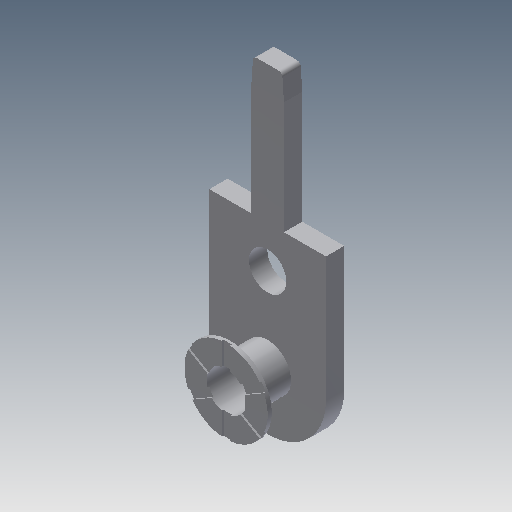
# Autodesk Inventor part: Part4_panel pot
Saved by Autodesk Inventor 2020 (Build 240168000, 168)
## iProperties
Created: 2016-08-22
Part Number: Part4_panel pot
Material: Generic
Document SubType Name: Modeling
Designer: Tom
Density: 1 g/cm^3
Appearance: Default
Author: Tom
Autodesk Inventor part; units mm, degrees
ref_plane "YZ Plane" through (0, 0, 0) normal (1, 0, 0) x (0, 1, 0)
ref_plane "XZ Plane" through (0, 0, 0) normal (0, 1, 0) x (-1, 0, 0)
ref_plane "XY Plane" through (0, 0, 0) normal (0, 0, 1) x (1, 0, 0)
sketch "Sketch1" plane through (0, 0, 0) normal (0, 0, 1) x (1, 0, 0)
  arc A0 (-1.778, 0) -> (1.778, 0) centre (0, 0) ccw
  line L0 (-1.778, 0) -> (-1.778, 3.81)
  line L1 (-1.778, 3.81) -> (1.778, 3.81)
  line L2 (1.778, 3.81) -> (1.778, 0)
  dimension "d0" = 3.556
  dimension "d1" = 3.81
  constraints: 6 end point, 2 point on circle, 2 tangent, 1 centre point, 1 coincident, 1 perpendicular, 1 vertical
  measures "d0" diameter of A0
  measures "d1" distance from line of L1 A0.centre
extrude "Extrusion1" add sketch "Sketch1" along normal blind 0.5588
hole "Hole1" at (0, 0, 0.5588) direction (0, 0, -1) diameter 1.143 end through all
sketch "Sketch3" plane through (0, 0, 0) normal (1, 0, 0) x (0, 1, 0)
  line L0 (-0.5908, 1.8288) -> (-1.27, 1.8288)
  line L1 (-1.27, 1.8288) -> (-1.27, 1.7018)
  line L2 (0, 0.5588) -> (-1.778, 0.5588) projected
  line L3 (0, 1.8288) -> (0, 0.5588)
  line L4 (-0.5908, 0.5588) -> (-0.5908, 1.8288)
  line L5 (-1.27, 1.7018) -> (-0.7178, 1.7018)
  line L6 (0.5715, 0) -> (-0.5715, 0) projected
  line L7 (-0.5715, 0.5588) -> (0.5715, 0.5588) projected
  line L8 (-0.7178, 1.7018) -> (-0.7178, 0.5588)
  line L9 (-0.7178, 0.5588) -> (-0.5908, 0.5588)
  point P0 (0, 0)
  dimension "d21" = 0.127
  dimension "d22" = 1.27
  constraints: 14 end point, 4 perpendicular, 2 point on line, 1 horizontal, 1 parallel
  measures "d21" distance from line of L4 L5.end
  measures "d22" distance from line of L3 L0.end
revolve "Revolution1" add sketch "Sketch3" angle 360 about axis through (0, 0, 1.8288) along (0, 0, -1)
sketch "Sketch4" plane through (0, 0, 1.8288) normal (0, 0, 1) x (1, 0, 0)
  circle A0 centre (0, 0) radius 1.27 projected
  line L0 (-0.127, 0.3054) -> (0.127, 0.3054)
  line L1 (0.127, 0.3054) -> (0.127, 1.3789)
  line L2 (0.127, 1.3789) -> (-0.127, 1.3789)
  line L3 (-0.127, 1.3789) -> (-0.127, 0.3054)
  line L4 (-0.328, 0.0427) -> (-0.201, 0.2627)
  line L5 (-0.201, 0.2627) -> (-1.1307, 0.7994)
  line L6 (-1.1307, 0.7994) -> (-1.2577, 0.5795)
  line L7 (-1.2577, 0.5795) -> (-0.328, 0.0427)
  line L8 (-0.201, -0.2627) -> (-0.328, -0.0427)
  line L9 (-0.328, -0.0427) -> (-1.2577, -0.5795)
  line L10 (-1.2577, -0.5795) -> (-1.1307, -0.7994)
  line L11 (-1.1307, -0.7994) -> (-0.201, -0.2627)
  line L12 (0.127, -0.3054) -> (-0.127, -0.3054)
  line L13 (-0.127, -0.3054) -> (-0.127, -1.3789)
  line L14 (-0.127, -1.3789) -> (0.127, -1.3789)
  line L15 (0.127, -1.3789) -> (0.127, -0.3054)
  line L16 (0.328, -0.0427) -> (0.201, -0.2627)
  line L17 (0.201, -0.2627) -> (1.1307, -0.7994)
  line L18 (1.1307, -0.7994) -> (1.2577, -0.5795)
  line L19 (1.2577, -0.5795) -> (0.328, -0.0427)
  line L20 (0.201, 0.2627) -> (0.328, 0.0427)
  line L21 (0.328, 0.0427) -> (1.2577, 0.5795)
  line L22 (1.2577, 0.5795) -> (1.1307, 0.7994)
  line L23 (1.1307, 0.7994) -> (0.201, 0.2627)
  dimension "d24" = 0.254
  dimension "d25" = 0.127
  dimension "d28" = 360
  constraints: 48 end point, 2 parallel, 1 horizontal, 1 perpendicular, 49 other
  measures "d24" distance between parallel lines of L3 L1
  measures "d25" horizontal distance of L0.end A0.centre
extrude "Extrusion2" cut sketch "Sketch4" against normal blind 0.0508 contours L21 L20 L23 A0 | A0 L23 L22 L21 | L19 L18 L17 A0 | A0 L17 L16 L19 | L1 L0 L3 A0 | A0 L3 L2 L1 | L15 L14 L13 A0 | A0 L13 L12 L15 | L5 L4 L7 A0 | A0 L7 L6 L5 | L11 L10 L9 A0 | A0 L9 L8 L11
sketch "Sketch5" plane through (0, 0, 0.5588) normal (0, 0, 1) x (1, 0, 0)
  arc A0 (-1.778, 0) -> (1.778, 0) centre (0, 0) ccw projected
  line L0 (1.778, 3.81) -> (-1.778, 3.81) projected
  line L1 (-0.4953, 3.81) -> (0.4953, 3.81)
  line L2 (0.4953, 3.81) -> (0.4953, 8.001)
  line L3 (0.4953, 8.001) -> (-0.4953, 8.001)
  line L4 (-0.4953, 8.001) -> (-0.4953, 3.81)
  dimension "d32" = 4.191
  dimension "d33" = 0.9906
  dimension "d34" = 0.4953
  constraints: 8 end point, 2 parallel, 1 horizontal, 1 perpendicular, 1 point on line
  measures "d32" distance of L3.end L1.start
  measures "d33" distance of L2.end L3.end
  measures "d34" horizontal distance of L1.end A0.centre
extrude "Extrusion3" add sketch "Sketch5" against normal up to surface (0.5588 mm away)
chamfer "Chamfer1" distance 0.0508 distance2 0.762 1 edges at (0.4953, 8.001, 0.2794) measured on face at (-0.0047, 8.001, 0.2794)
chamfer "Chamfer2" distance 0.762 distance2 0.0508 1 edges at (-0.4953, 8.001, 0.2794) measured on face at (-0.4953, 7.501, 0.2794)
fillet "Fillet2" radius 0.127 2 edges at (0.4445, 8.001, 0.2794) (-0.4445, 8.001, 0.2794)
sketch "Sketch6" plane through (0, 0, 0) normal (0, 0, -1) x (-1, 0, 0)
  arc A0 (-1.778, 0) -> (1.778, 0) centre (0, 0) ccw projected
  point P0 (0, 2.54)
  dimension "d45" = 2.54
  measures "d45" distance of point (0, 2.54) A0.centre
hole "Hole2" at (0, 2.54, 0) direction (0, 0, 1) diameter 1.143 end through all
equation "\"d25\" = 0.5 * d24"
equation "\"d34\" = 0.5 * d33"
body "Solid1"
